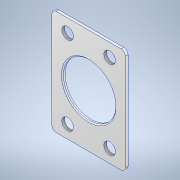
# Autodesk Inventor part: Прокладка крейцкопф_CPY
Saved by Autodesk Inventor 2021 (Build 250183000, 183)
## iProperties
Created: 2020-12-02
Part Number: Прокладка крейцкопф_CPY
Material: Алюминий 6061
Document SubType Name: Modeling
Designer: Тимоха
Mass: 155.66 g
Surface Area: 276.361 cm^2
Volume: 57.652 cm^3
Density: 2.7 g/cm^3
Appearance: Алюминий — плоский
Author: Тимоха
Autodesk Inventor part; units mm, degrees
ref_plane "YZ Plane" through (0, 0, 0) normal (1, 0, 0) x (0, 1, 0)
ref_plane "XZ Plane" through (0, 0, 0) normal (0, 1, 0) x (-1, 0, 0)
ref_plane "РабПлоскость1" through (0, 0, 0) normal (0, 0, 1) x (1, 0, 0)
sketch "Эскиз1" plane through (0, 0, 0) normal (0, 0, 1) x (1, 0, 0)
  circle A0 centre (0, 0) radius 50 projected
  line L0 (-70, -92) -> (-70, 92)
  line L1 (-62, 100) -> (62, 100)
  line L2 (70, 92) -> (70, -92)
  line L3 (62, -100) -> (-62, -100)
  line L4 (-70, -100) -> (70, 100) construction
  line L5 (-70, 100) -> (70, -100) construction
  arc A1 (-62, 100) -> (-70, 92) centre (-62, 92) ccw
  arc A2 (70, 92) -> (62, 100) centre (62, 92) ccw
  arc A3 (62, -100) -> (70, -92) centre (62, -92) ccw
  arc A4 (-70, -92) -> (-62, -100) centre (-62, -92) ccw
  line L6 (0, 75) -> (-40, 75)
  line L7 (-40, 75) -> (40, 75)
  line L8 (40, 75) -> (40, -75)
  line L9 (40, -75) -> (-40, -75)
  line L10 (-40, -75) -> (-40, 75)
  circle A5 centre (-40, 75) radius 11
  circle A6 centre (40, 75) radius 11
  circle A7 centre (40, -75) radius 11
  circle A8 centre (-40, -75) radius 11
  point P0 (0, 0)
  dimension "d8" = 200
  dimension "d9" = 140
  dimension "d10" = 8
  dimension "d11" = 8
  dimension "d12" = 8
  dimension "d13" = 8
  dimension "d14" = 40
  dimension "d15" = 80
  dimension "d16" = 150
  dimension "d17" = 22
  dimension "d18" = 22
  dimension "d19" = 22
  dimension "d20" = 22
  constraints: 22 end point, 8 centre point, 8 point on circle, 8 point on line, 8 tangent, 4 coincident, 4 parallel, 2 horizontal, 2 midpoint, 2 perpendicular
  measures "d8" distance of L4.start L5.start
  measures "d9" distance of L5.start L4.end
  measures "d10" radius of A1
  measures "d11" radius of A2
  measures "d12" radius of A3
  measures "d13" radius of A4
  measures "d14" distance of L6.start L6.end
  measures "d15" distance of L8.end L9.end
  measures "d16" distance of L7.end L8.end
  measures "d17" diameter of A5
  measures "d18" diameter of A6
  measures "d19" diameter of A7
  measures "d20" diameter of A8
extrude "Выдавливание1" add sketch "Эскиз1" along normal blind 5 contours A0 L10 A5 L6 L7 A6 L8 | L8 A7 L9 A8 L10 A0 | L0 A1 L1 A2 L2 A3 L3 A4
chamfer "Фаска1" distance 2 angle 45 1 edges at (-50, 0, 5)
